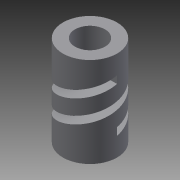
# Autodesk Inventor part: z-coupler
Saved by Autodesk Inventor 2013 (Build 170138000, 138)
## iProperties
Created: 2014-01-26
Part Number: z-coupler
Material: Generic
Document SubType Name: Modeling
Designer: Masta
Density: 1 g/cm^3
Author: Masta
Autodesk Inventor part; units mm, degrees
ref_plane "YZ Plane" through (0, 0, 0) normal (1, 0, 0) x (0, 1, 0)
ref_plane "XZ Plane" through (0, 0, 0) normal (0, 1, 0) x (-1, 0, 0)
ref_plane "XY Plane" through (0, 0, 0) normal (0, 0, 1) x (1, 0, 0)
sketch "Sketch1" plane through (0, 0, 0) normal (0, 0, 1) x (1, 0, 0)
  circle A0 centre (0, 0) radius 9
  circle A1 centre (0, 0) radius 2.5
  dimension "d0" = 18
  dimension "d3" = 5
  constraints: 2 centre point, 2 coincident
  measures "d0" diameter of A0
  measures "d3" diameter of A1
extrude "Extrusion1" add sketch "Sketch1" along normal blind 30
sketch "Sketch2" plane through (0, 0, 30) normal (0, 0, 1) x (1, 0, 0)
  circle A0 centre (0, 0) radius 2.5 projected
  circle A1 centre (0, 0) radius 9 projected
  circle A2 centre (0, 0) radius 5
  dimension "d4" = 10
  constraints: 1 centre point, 1 coincident
  measures "d4" diameter of A2
extrude "Extrusion2" cut sketch "Sketch2" against normal blind 20 contours A2
sketch "Sketch3" plane through (0, 0, 0) normal (0, 1, 0) x (-1, 0, 0)
  line L0 (9, 30) -> (9, 0) projected
  line L1 (9, 0) -> (2.5, 0) projected
  line L2 (2.5, 0) -> (2.5, 10) projected
  line L3 (2.5, 10) -> (5, 10) projected
  line L4 (5, 10) -> (5, 30) projected
  line L5 (5, 30) -> (9, 30) projected
  line L6 (-9, 0) -> (-9, 30) projected
  line L7 (-9, 30) -> (-5, 30) projected
  line L8 (-5, 30) -> (-5, 10) projected
  line L9 (-5, 10) -> (-2.5, 10) projected
  line L10 (-2.5, 10) -> (-2.5, 0) projected
  line L11 (-2.5, 0) -> (-9, 0) projected
  line L12 (0, 0) -> (9, 0)
  line L13 (9, 0) -> (9, 30)
  line L14 (9, 30) -> (0, 30)
  line L15 (0, 30) -> (0, 0)
  line L16 (-9, 6.25) -> (-5, 6.25)
  line L17 (-5, 6.25) -> (-5, 8.75)
  line L18 (-5, 8.75) -> (-9, 8.75)
  line L19 (-9, 8.75) -> (-9, 6.25)
  line L20 (-9, 15) -> (0, 15) construction
  line L21 (-9, 7.5) -> (-5, 7.5) construction
  dimension "d20" = 2.5
  dimension "d22" = 7.5
  constraints: 20 end point, 4 midpoint, 4 parallel, 2 horizontal, 2 perpendicular, 2 point on line
  measures "d20" distance between parallel lines of L16 L18
  measures "d22" distance between parallel lines of L21 L20
extrude "Extrusion3" [suppressed]
coil "Coil1" sketch "Sketch3" operation cut axis through (0, 0, -10) along (0, 0, 1) pitch 15 turns 1 hand right contours L6 L18 L17 L16
pattern_circular "Circular Pattern1" count 2 over 360 about axis through (0, 0, -10) along (0, 0, 1) of "Coil1"
body "Solid1"
